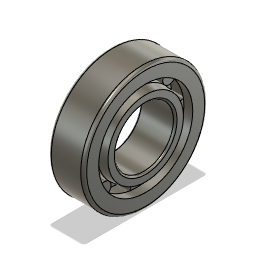
Bearing_GOST_8328-75_32000 (Autodesk Fusion 360 design; units mm, degrees)
Autodesk Fusion 360 part; units mm, degrees
sketch "Sketch1" plane through (0, 0, 0) normal (0, 0, 1) x (1, 0, 0)
  line L0 (-32.0679, 0) -> (32.0679, 0)
  line L1 (-6, 10) -> (6, 10)
  line L2 (6, 10) -> (6, 12.771)
  line L3 (6, 12.771) -> (3, 13.3)
  line L4 (3, 13.3) -> (-3, 13.3)
  line L5 (-3, 13.3) -> (-6, 12.771)
  line L6 (-6, 12.771) -> (-6, 10)
  line L7 (-3, 15.93) -> (-3, 17.7)
  line L8 (-3, 17.7) -> (3, 17.7)
  line L9 (3, 17.7) -> (3, 15.93)
  line L10 (3, 15.93) -> (6, 15.93)
  line L11 (6, 15.93) -> (6, 21)
  line L12 (6, 21) -> (-6, 21)
  line L13 (-6, 21) -> (-6, 15.93)
  line L14 (-6, 15.93) -> (-3, 15.93)
  line L15 (-3, 15.93) -> (-3, 13.3)
  line L16 (3, 15.93) -> (3, 13.3)
  line L17 (0, 17.7) -> (0, 13.3) construction
  line L18 (-3, 15.5) -> (3, 15.5)
  point P0 (0, 10)
  point P1 (0, 15.5)
  dimension "d2" = 10
  dimension "d3" = 12
  dimension "d4" = 20
  dimension "d5" = 26.6
  dimension "d6" = 3
  dimension "d7" = 42
  dimension "d8" = 35.4
  dimension "d17" = 31.86
  constraint horizontal L0
  constraint midpoint L0 origin
  constraint horizontal L1
  constraint perpendicular L1 L2
  constraint perpendicular L2 L4
  constraint perpendicular L1 L6
  constraint equal L3 L5
  constraint equal L2 L6
  constraint midpoint L1 P0
  constraint vertical origin P0
  constraint vertical L7
  constraint perpendicular L7 L8
  constraint perpendicular L8 L9
  constraint perpendicular L9 L10
  constraint perpendicular L10 L11
  constraint perpendicular L11 L12
  constraint perpendicular L12 L13
  constraint perpendicular L13 L14
  constraint equal L11 L13
  constraint equal L10 L14
  constraint vertical L3.end L9.end
  constraint vertical L2.end L10.end
  constraint vertical L5.end L13.end
  constraint midpoint L8 L17.start
  constraint midpoint L4 L17.end
  constraint coincident L15 L18.start
  constraint coincident L16 L18.end
  constraint perpendicular L16 L18
  constraint midpoint L17 P1
  constraint coincident L18 P1
  measures "d2" angle of L3 L4
  measures "d3" distance of L2 L6
  measures "d6" horizontal distance of L1.end L3.end
revolve "Revolve1" add sketch "Sketch1" angle 360 about axis through (-32.0679, 0, 0) along (1, 0, 0) contours L1 L2 L3 L4 L5 L6 | L7 L8 L9 L10 L11 L12 L13 L14 makes body 1 at (2, 20.9739, -1.0468) makes body 2 at (-2, 9.9876, -0.4985)
revolve "Revolve2" add sketch "Sketch1" angle 360 about axis through (-3, 15.5, 0) along (1, 0, 0) separate body contours L7 L8 L9 L15 L16 L18 makes body 3
pattern_circular "C-Pattern1" count 8 over 360 about axis through (-32.0679, 0, 0) along (1, 0, 0) of bodies 3 makes body 4 at (1, 12.663, 12.3532) makes body 5 at (1, 0.219, 17.6891) makes body 6 at (1, -12.3532, 12.663) makes body 7 at (1, -17.6891, 0.219) makes body 8 at (1, -12.663, -12.3532) makes body 9 at (1, -0.219, -17.6891) makes body 10 at (1, 12.3532, -12.663)
fillet "Fillet1" radius 1 2 edges at (-6, -7.5939, 19.5789) (6, -7.5939, 19.5789) on bodies 1
fillet "Fillet2" radius 0.6 2 edges at (-6, -3.6162, 9.3233) (6, -3.6162, 9.3233) on bodies 2
